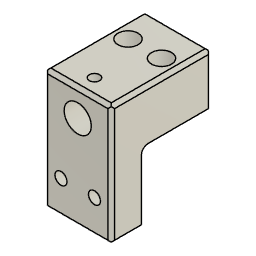
y-rod-holder (Autodesk Fusion 360 design; units mm, degrees)
Autodesk Fusion 360 part; units mm, degrees
sketch "Sketch1" plane through (0, 0, 0) normal (0, 1, 0) x (1, 0, 0)
  line L0 (10, 10) -> (-10, 10)
  line L1 (-10, 10) -> (-10, -10)
  line L2 (-10, -10) -> (10, -10)
  line L3 (10, -10) -> (10, 10)
  line L4 (10, 10) -> (-10, -10) construction
  line L5 (-10, 10) -> (10, -10) construction
  circle A0 centre (-5, 0) radius 1.8
  circle A1 centre (5, 0) radius 1.8
  line L6 (-10, -10) -> (10, -10)
  line L7 (10, -10) -> (10, -26)
  line L8 (10, -26) -> (-10, -26)
  line L9 (-10, -26) -> (-10, -10)
  line L10 (10, -10) -> (-10, -26) construction
  line L11 (-10, -10) -> (10, -26) construction
  circle A2 centre (0, -18) radius 4.05
  dimension "d52" = 20
  dimension "d53" = 20
  dimension "d55" = 10
  dimension "d56" = 3.6
  dimension "d57" = 3.6
  dimension "d58" = 20
  dimension "d59" = 16
  dimension "d60" = 8.1
  constraint horizontal L0
  constraint perpendicular L0 L1
  constraint parallel L0 L2
  constraint parallel L1 L3
  constraint coincident L4 origin
  constraint coincident L5 origin
  constraint horizontal L6
  constraint vertical L7
  constraint horizontal L8
  constraint vertical L9
  constraint midpoint L11 A2.centre
  measures "d52" distance of L1.end L2.end
  measures "d53" distance of L0.end L1.end
  measures "d55" distance of A0.centre A1.centre
  measures "d56" diameter of A0
  measures "d57" diameter of A1
  measures "d58" distance of L1.end L2.end
  measures "d59" distance of L1.end L8.end
  measures "d60" diameter of A2
extrude "Extrude1" add sketch "Sketch1" against normal blind 10
extrude "Extrude2" add sketch "Sketch1" along normal blind 20 contours L2 L6 L7 L8 L9 | A2
sketch "Sketch2" plane through (0, 0, 26) normal (0, 0, 1) x (-1, 0, 0)
  line L0 (10, -20) -> (-10, -20)
  line L1 (-10, -20) -> (-10, 0)
  line L2 (-10, 0) -> (10, 0)
  line L3 (10, 0) -> (10, -20)
  line L4 (-10, 0) -> (10, -20) construction
  line L5 (10, 0) -> (-10, -20) construction
  circle A0 centre (5, -10) radius 1.8
  circle A1 centre (-5, -10) radius 1.8
  line L6 (10, -20) -> (10, 10)
  line L7 (10, 10) -> (-10, 10)
  line L8 (-10, 10) -> (-10, -20)
  line L9 (-10, -20) -> (10, -20)
  line L10 (10, 0) -> (-10, 10) construction
  line L11 (-10, 0) -> (10, 10) construction
  circle A2 centre (0, 5) radius 1.55
  circle A3 centre (-5, -10) radius 3
  circle A4 centre (5, -10) radius 3
  dimension "d65" = 20
  dimension "d66" = 20
  dimension "d68" = 10
  dimension "d69" = 3.6
  dimension "d70" = 3.6
  dimension "d82" = 3.1
  dimension "d89" = 6
  dimension "d90" = 6
  constraint horizontal L0
  constraint vertical L1
  constraint horizontal L2
  constraint vertical L3
  constraint coincident L7.end L8.start
  constraint coincident L6.end L7.start
  constraint midpoint L11 A2.centre
  constraint concentric A1 A3
  constraint concentric A0 A4
  measures "d65" distance of L0.start L0.end
  measures "d66" distance of L0.start L2.end
  measures "d68" distance of A0.centre A1.centre
  measures "d69" diameter of A0
  measures "d70" diameter of A1
  measures "d82" diameter of A2
  measures "d89" diameter of A3
  measures "d90" diameter of A4
extrude "Extrude6" cut sketch "Sketch2" against normal blind 16 contours A0 | A1
extrude "Extrude7" cut sketch "Sketch2" against normal blind 4.5 contours A2
fillet "Fillet2" radius 1 1 edges at (0, 0, 10)
extrude "Extrude8" cut sketch "Sketch2" against normal blind 6 contours A3 | A4
chamfer "Chamfer4" distance 1 angle 45 19 edges at (10, 20, 18) (10, 10.5, 10) (10, 0, -0.5) (10, 0.2929, 9.7071) (10, 5, 26) (0, 20, 26) (-10, 5, 26) (0, -10, 26) (10, -10, 8) (-10, 0, -0.5) (-10, 0.2929, 9.7071) (-10, 10.5, 10) (-10, 20, 18) (0, 20, 10) (0, 0, -10) (10, -5, -10) (-10, -5, -10) (0, -10, -10) (-10, -10, 8)
named bodies: "holder"
